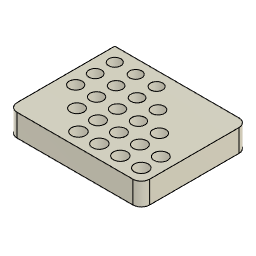
M3 Het Set Insert Parameter Block (Autodesk Fusion 360 design; units mm, degrees)
Autodesk Fusion 360 part; units mm, degrees
sketch "Sketch1" plane through (0, 0, 0) normal (0, 0, 1) x (1, 0, 0)
  line L0 (0, 0) -> (47.5, 0)
  line L1 (47.5, 0) -> (47.5, 38)
  circle A0 centre (5, 33) radius 2.175
  line L2 (5, 33) -> (5, 26) construction
  circle A1 centre (5, 26) radius 2.25
  circle A2 centre (12.5, 26) radius 2.25
  circle A3 centre (12.5, 33) radius 2.175
  circle A4 centre (20, 26) radius 2.25
  circle A5 centre (20, 33) radius 2.175
  line L3 (5, 26) -> (5, 19) construction
  line L4 (5, 19) -> (5, 12) construction
  circle A6 centre (5, 19) radius 2.325
  circle A7 centre (5, 12) radius 2.4
  circle A8 centre (12.5, 19) radius 2.325
  circle A9 centre (12.5, 12) radius 2.4
  circle A10 centre (20, 19) radius 2.325
  circle A11 centre (20, 12) radius 2.4
  circle A12 centre (27.5, 26) radius 2.25
  circle A13 centre (27.5, 33) radius 2.175
  circle A14 centre (27.5, 19) radius 2.325
  circle A15 centre (27.5, 12) radius 2.4
  circle A16 centre (35, 26) radius 2.25
  circle A17 centre (35, 33) radius 2.175
  circle A18 centre (35, 19) radius 2.325
  circle A19 centre (35, 12) radius 2.4
  line L5 (5, 12) -> (5, 5) construction
  circle A20 centre (5, 5) radius 2.475
  circle A21 centre (12.5, 5) radius 2.475
  circle A22 centre (20, 5) radius 2.475
  circle A23 centre (27.5, 5) radius 2.475
  circle A24 centre (35, 5) radius 2.475
  circle A25 centre (42.5, 26) radius 2.25
  circle A26 centre (42.5, 33) radius 2.175
  circle A27 centre (42.5, 19) radius 2.325
  circle A28 centre (42.5, 12) radius 2.4
  circle A29 centre (42.5, 5) radius 2.475
  line L6 (47.5, 38) -> (0, 38)
  line L7 (0, 38) -> (0, 0)
  dimension "d2" = 4.35
  dimension "d4" = 4.5
  dimension "d7" = 7.5
  dimension "d8" = 0
  dimension "d13" = 4.65
  dimension "d14" = 4.8
  dimension "d21" = 4.95
  dimension "d27" = 5
  dimension "d28" = 5
  dimension "d29" = 5
  dimension "d30" = 5
  constraint horizontal L0
  constraint vertical L1
  constraint coincident L0.start L7.end
  constraint coincident A0.centre L2.start
  constraint coincident L2.end A1.centre
  constraint parallel L2 L3
  constraint parallel L3 L4
  constraint coincident L3.end L4.start
  constraint coincident L4.end A7.centre
  constraint parallel L4 L5
  constraint coincident L5.end A20.centre
  constraint horizontal L6
  constraint vertical L7
  measures "d2" diameter of A0
  measures "d4" diameter of A1
  measures "d13" diameter of A6
  measures "d14" diameter of A7
  measures "d21" diameter of A20
  measures "d27" distance of L1 A26.centre
  measures "d28" distance of A0.centre L7
  measures "d29" distance of A26.centre L6
  measures "d30" distance of L0 A29.centre
sketch "Sketch2" plane through (0, 0, 0) normal (0, 0, 1) x (1, 0, 0)
  line L0 (47.5, 0) -> (47.5, 38)
  line L1 (0, 0) -> (47.5, 0)
  line L2 (47.5, 38) -> (0, 38)
  line L3 (0, 38) -> (0, 0)
extrude "Extrude1" add sketch "Sketch2" against normal blind 8
extrude "Extrude2" cut sketch "Sketch1" against normal blind 5.8 contours A0 | A1 | A6
extrude "Extrude3" cut sketch "Sketch1" against normal blind 5.8 draft -2 contours A2 | A3 | A8 | A9
extrude "Extrude4" cut sketch "Sketch1" against normal blind 5.7 draft -4 contours A4 | A5 | A10 | A11 | A22
extrude "Extrude5" cut sketch "Sketch1" against normal blind 5.8 draft -6 contours A12 | A14 | A15 | A23
extrude "Extrude6" cut sketch "Sketch1" against normal blind 5.8 draft -8 contours A18 | A19 | A24
extrude "Extrude7" cut sketch "Sketch1" against normal blind 5.8 draft -10 contours A28 | A29
fillet "Fillet1" radius 3 3 edges at (0, 0, -4) (47.5, 0, -4) (47.5, 38, -4)
equation "d11 = -extrude_depth"
equation "d15 = -extrude_depth"
equation "d19 = -extrude_depth"
equation "d22 = -extrude_depth"
equation "d24 = -extrude_depth"
equation "extrude_depth = 5.8 mm"
